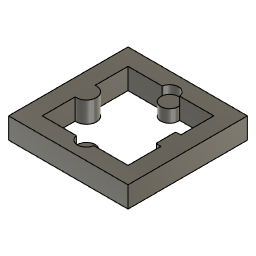
grove_1x1_sensor_mount (Autodesk Fusion 360 design; units mm, degrees)
Autodesk Fusion 360 part; units mm, degrees
sketch "Sketch1" plane through (0, 0, 0) normal (0, 0, 1) x (1, 0, 0)
  line L0 (14.2, -14.2) -> (-14.2, -14.2)
  line L1 (-14.2, -14.2) -> (-14.2, 14.2)
  line L2 (-14.2, 14.2) -> (14.2, 14.2)
  line L3 (14.2, 14.2) -> (14.2, -14.2)
  line L4 (14.2, -14.2) -> (-14.2, 14.2) construction
  line L5 (-14.2, -14.2) -> (14.2, 14.2) construction
  dimension "d1" = 28.4
  dimension "d2" = 28.4
  constraint horizontal L0
  constraint perpendicular L0 L1
  constraint parallel L0 L2
  constraint parallel L1 L3
  constraint coincident L4 origin
  constraint coincident L5 origin
  measures "d1" distance of L1.end L2.end
  measures "d2" distance of L0 L2
extrude "Extrude1" add sketch "Sketch1" along normal blind 5
shell "Shell1" thickness 4 removed faces 2 at (-4.7333, 4.7333, 5) at (-4.7333, 4.7333, 0)
sketch "Sketch2" plane through (0, 0, 5) normal (0, 0, 1) x (-1, 0, 0)
  line L0 (-10.2, -10.2) -> (-10.2, 10.2)
  line L1 (-10.2, 10.2) -> (10.2, 10.2)
  line L2 (10.2, 10.2) -> (10.2, -10.2)
  line L3 (10.2, -10.2) -> (-10.2, -10.2)
  line L4 (-14.2, -14.2) -> (14.2, -14.2)
  line L5 (14.2, -14.2) -> (14.2, 14.2)
  line L6 (14.2, 14.2) -> (-14.2, 14.2)
  line L7 (-14.2, 14.2) -> (-14.2, -14.2)
  circle A0 centre (0, -9.9) radius 2.1
  circle A1 centre (-9.9, 0) radius 2.4
  line L8 (-10.2, 0) -> (10.2, 0) construction
  line L9 (0, -10.2) -> (0, 10.2) construction
  circle A2 centre (0, 9.9) radius 2.1
  circle A3 centre (9.9, 0) radius 2.4
  line L10 (-9, -2.2249) -> (-9, 2.2249)
  dimension "d11" = 4.2
  dimension "d12" = 0.3
  dimension "d14" = 4.8
  dimension "d15" = 0.3
  dimension "d18" = 4.2
  dimension "d19" = 0.3
  dimension "d21" = 4.8
  dimension "d31" = 0.3
  dimension "d33" = 0.9
  constraint midpoint L0 L8.start
  constraint midpoint L2 L8.end
  constraint midpoint L3 L9.start
  constraint midpoint L1 L9.end
  constraint coincident A0.centre L9
  constraint coincident L9 A2.centre
  constraint coincident L8 A3.centre
  constraint coincident A1 L10.start
  constraint coincident A1 L10.end
  constraint perpendicular L8 L10
  measures "d11" diameter of A0
  measures "d12" distance of L3 A0.centre
  measures "d14" diameter of A1
  measures "d15" distance of L0 A1.centre
  measures "d18" diameter of A2
  measures "d19" distance of L1 A2.centre
  measures "d21" diameter of A3
  measures "d31" distance of L2 A3.centre
  measures "d33" distance of A1.centre L10
extrude "Extrude2" add sketch "Sketch2" against normal blind 5 contours L0 A1 L10 | L2 A3 picked at (9.4042, -0.3949)
extrude "Extrude3" cut sketch "Sketch2" against normal blind 2 contours L3 A0 | L1 A2 picked at (0.357, -10.7865) picked at (0.0996, 10.7929)
extrude "Extrude4" add sketch "Sketch2" against normal blind 3 from surface at -2 contours L3 A0 | L1 A2 picked at (0.2572, -9.449) picked at (0.2572, 9.449)
